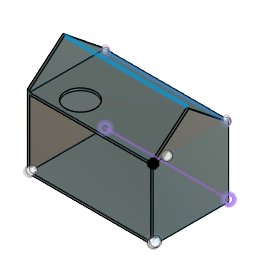
Haus SH (Autodesk Fusion 360 design; units mm, degrees)
part number: 2026-08-06-17-03-33-858
Autodesk Fusion 360 part; units mm, degrees
sketch "Sketch1" plane through (0, 0, 0) normal (0, 0, 1) x (1, 0, 0)
  line L0 (0, 0) -> (275, 0)
  line L1 (275, 0) -> (275, -165)
  line L2 (275, -165) -> (0, -165)
  line L3 (0, -165) -> (0, 0)
  dimension "d1" = 275
  dimension "d2" = 165
  constraint horizontal L0
  constraint vertical L1
  constraint horizontal L2
  constraint vertical L3
  constraint coincident L0.start L3.end
  measures "d1" distance of L0.start L0.end
  measures "d2" distance of L0.start L2.end
extrude "Extrude1" add sketch "Sketch1" along normal blind 5
sketch "Sketch2" plane through (0, 0, 5) normal (0, 0, 1) x (-1, 0, 0)
  line L0 (0, 165) -> (-275, 165)
  line L1 (-275, 165) -> (-275, 0)
  line L2 (-275, 0) -> (0, 0)
  line L3 (0, 0) -> (0, 165)
  line L4 (0, 0) -> (-275, 0)
  line L5 (-275, 0) -> (-275, 5)
  line L6 (-275, 5) -> (0, 5)
  line L7 (0, 5) -> (0, 0)
  line L8 (-275, 0) -> (-270, 0)
  line L9 (-270, 0) -> (-270, 165)
  line L10 (-270, 165) -> (-275, 165)
  line L11 (-275, 165) -> (-275, 0)
  line L12 (-275, 165) -> (0, 165)
  line L13 (0, 165) -> (0, 160)
  line L14 (0, 160) -> (-275, 160)
  line L15 (-275, 160) -> (-275, 165)
  line L16 (0, 0) -> (-5, 0)
  line L17 (-5, 0) -> (-5, 165)
  line L18 (-5, 165) -> (0, 165)
  line L19 (0, 165) -> (0, 0)
  dimension "d5" = 5
  dimension "d6" = 5
  dimension "d7" = 165
  dimension "d8" = 275
  dimension "d9" = 5
  dimension "d10" = 165
  constraint horizontal L4
  constraint vertical L5
  constraint horizontal L6
  constraint vertical L7
  constraint coincident L2.end L3.start
  constraint horizontal L8
  constraint vertical L9
  constraint horizontal L10
  constraint vertical L11
  constraint coincident L1.end L2.start
  constraint horizontal L12
  constraint vertical L13
  constraint horizontal L14
  constraint vertical L15
  constraint coincident L0.end L1.start
  constraint horizontal L16
  constraint vertical L17
  constraint horizontal L18
  constraint vertical L19
  measures "d5" distance of L2.end L6.end
  measures "d6" distance of L1.end L8.end
  measures "d7" distance of L1.end L0.end
  measures "d8" distance of L0.end L0.start
  measures "d9" distance of L0.end L14.end
  measures "d10" distance of L2.end L0.start
sketch "Sketch3" plane through (0, 0, 5) normal (0, 0, 1) x (-1, 0, 0)
extrude "Extrude2" add sketch "Sketch2" along normal blind 150 contours L0 L3 L12 L13 L14 L17 L18 L19 | L3 L6 L14 L17 L19 | L2 L3 L4 L6 L7 L16 L17 L19
sketch "Sketch4" plane through (0, 0, 5) normal (0, 0, 1) x (-1, 0, 0)
  line L0 (-5, 0) -> (-5, 165)
  line L1 (-5, 165) -> (-275, 165)
  line L2 (-275, 165) -> (-275, 0)
  line L3 (-275, 0) -> (-5, 0)
sketch "Sketch5" plane through (0, 0, 5) normal (0, 0, 1) x (-1, 0, 0)
  line L0 (-275, 0) -> (-270, 0)
  line L1 (-270, 0) -> (-270, 165)
  line L2 (-270, 165) -> (-275, 165)
  line L3 (-275, 165) -> (-275, 0)
  line L4 (-5, 0) -> (-5, 165)
  dimension "d13" = 5
  dimension "d14" = 165
  dimension "d15" = 270
  constraint horizontal L0
  constraint vertical L1
  constraint horizontal L2
  constraint vertical L3
  measures "d13" distance of L0.start L0.end
  measures "d14" distance of L0.start L2.end
  measures "d15" distance of L3 L4
extrude "Extrude3" add sketch "Sketch5" along normal blind 150
sketch "Sketch6" plane through (0, 0, 0) normal (0, 1, 0) x (1, 0, 0)
  line L0 (269.7146, -155) -> (269.7146, -150)
  line L1 (4.7146, -150) -> (4.7146, -155)
  line L2 (5, -5) -> (275, -5)
  dimension "d19" = 5
  constraint vertical L0
  constraint vertical L1
  measures "d19" distance of L1.end L1.start
sketch "Sketch7" plane through (0, 0, 5) normal (0, 0, 1) x (-1, 0, 0)
  line L0 (-5.2103, 3.9572, 144.946) -> (-270.2103, 3.9572, 144.946)
  line L1 (-270.2103, 3.9572, 144.946) -> (-270.2103, 3.9573, 149.9988)
  line L2 (-270.2103, 3.9573, 149.9988) -> (-5.2104, 3.9572, 149.946)
  line L3 (-5.2104, 3.9572, 149.946) -> (-5.2103, 3.9572, 144.946)
  line L4 (-275, 165) -> (-275, 160)
  line L5 (-275, 165) -> (-275, 160)
  line L6 (-5, 160) -> (-5, 165)
  line L7 (-5, 0) -> (-275, 0)
  dimension "d21" = 265
  dimension "d22" = 5
  dimension "d25" = 270
  dimension "d26" = 145
  dimension "d27" = 265
  constraint vertical L4
  constraint vertical L5
  constraint vertical L6
  measures "d25" distance of L6.end L4.start
sketch "Sketch8" plane through (0, 0, 0) normal (0, 1, 0) x (1, 0, 0)
  line L0 (5.2103, -149.946) -> (270.2103, -149.946)
  line L1 (5, -5) -> (275, -5)
sketch "Sketch9" plane through (0, 0, 5) normal (0, 0, 1) x (1, 0, 0)
sketch "Sketch10" plane through (275, 0, 0) normal (1, 0, 0) x (0, 1, 0)
  line L0 (-165, 0) -> (0, 0)
  line L1 (0, 0) -> (0, 155)
  line L2 (0, 155) -> (-165, 155)
  line L3 (-165, 155) -> (-165, 0)
  line L4 (-165, 155) -> (0, 155)
  line L5 (0, 155) -> (0, 150)
  line L6 (0, 150) -> (-165, 150)
  line L7 (-165, 150) -> (-165, 155)
  dimension "d29" = 165
  dimension "d30" = 5
  constraint horizontal L4
  constraint vertical L5
  constraint horizontal L6
  constraint vertical L7
  constraint coincident L2.end L3.start
  measures "d29" distance of L2.end L1.end
  measures "d30" distance of L2.end L6.end
extrude "Extrude4" add sketch "Sketch10" against normal blind 275 contours L1 L2 L3 L4 L5 L6 L7
sketch "Sketch11" plane through (0, 0, 0) normal (0, 1, 0) x (1, 0, 0)
sketch "Sketch12" plane through (0, 0, 0) normal (0, 1, 0) x (1, 0, 0)
sketch "Sketch13" plane through (275, 0, 0) normal (1, 0, 0) x (0, 1, 0)
  line L0 (-165, 155) -> (-165, 0)
  line L1 (-165, 0) -> (0, 0)
  line L2 (0, 0) -> (0, 155)
  line L3 (0, 155) -> (-165, 155)
  line L4 (-165, 155) -> (-135, 155) construction
  constraint horizontal L4
  constraint coincident L0.start L3.end
sketch "Sketch14" plane through (275, 0, 0) normal (1, 0, 0) x (0, 1, 0)
  line L0 (-170, 155) -> (-5, 155)
  line L1 (-5, 155) -> (-5, 225)
  line L2 (-5, 225) -> (-170, 225)
  line L3 (-170, 225) -> (-170, 155)
  line L4 (-165, 5) -> (0, 5)
  line L5 (-170, 155) -> (-87.1175, 224.5467)
  line L6 (-170, 155) -> (-61.8046, 155) construction
  line L7 (-87.1175, 224.5467) -> (13.9338, 144.1668)
  line L8 (-87.1175, 224.5467) -> (42.0037, 224.5467) construction
  dimension "d35" = 165
  dimension "d36" = 70
  dimension "d37" = 150
  dimension "d38" = 40
  dimension "d39" = 38.5
  constraint horizontal L0
  constraint vertical L1
  constraint horizontal L2
  constraint vertical L3
  constraint horizontal L6
  constraint horizontal L8
  measures "d35" distance of L0.start L0.end
  measures "d36" distance of L0.start L2.end
  measures "d37" distance of L0 L4
  measures "d38" angle of L5 L6
  measures "d39" angle of L7 L8
extrude "Extrude5" add sketch "Sketch14" against normal blind 5 contours L0 L1 L5 L7
sketch "Sketch15" plane through (0, 0, 155) normal (0, 0, 1) x (-1, 0, 0)
  line L0 (-270, 5) -> (-275, 5)
  line L1 (-275, 5) -> (-275, 0)
  line L2 (-275, 0) -> (0, 0)
  line L3 (0, 0) -> (0, 165)
  line L4 (0, 165) -> (-270, 165)
  line L5 (-270, 165) -> (-270, 5)
sketch "Sketch16" plane through (0, 0, 0) normal (-1, 0, 0) x (0, -1, 0)
  line L0 (0, 155) -> (0, 0)
  line L1 (0, 0) -> (165, 0)
  line L2 (165, 0) -> (165, 155)
  line L3 (165, 155) -> (0, 155)
  line L4 (0, 155) -> (87.0576, 225.2184)
  line L5 (87.0576, 225.2184) -> (165, 159.0254)
  line L6 (165, 159.0254) -> (165, 155)
  constraint coincident L0.start L3.end
  constraint coincident L2.end L3.start
  constraint perpendicular L3 L6
extrude "Extrude6" add sketch "Sketch16" against normal blind 5 contours L3 L4 L5 L6
sketch "Sketch17" plane through (5, 0, 0) normal (1, 0, 0) x (0, 1, 0)
  line L0 (-87.0576, 225.2184) -> (-165, 159.0254)
  line L1 (-165, 159.0254) -> (-165, 155)
  line L2 (-165, 155) -> (0, 155)
  line L3 (0, 155) -> (-87.0576, 225.2184)
sketch "Sketch18" plane through (0, 0, 0) normal (0, 1, 0) x (1, 0, 0)
  line L0 (5, -225.2184, -87.0576) -> (270, -225.2184, -87.0576)
  line L1 (270, -225.2184, -87.0576) -> (270, -220.2184, -87.0576)
  line L2 (270, -220.2184, -87.0576) -> (5, -220.2184, -87.0576)
  line L3 (5, -220.2184, -87.0576) -> (5, -225.2184, -87.0576)
  dimension "d44" = 265
  dimension "d45" = 5
sketch "Sketch19" plane through (275, 0, 0) normal (1, 0, 0) x (0, 1, 0)
  line L0 (-165, 155) -> (-165, 0)
  line L1 (-165, 0) -> (0, 0)
  line L2 (0, 0) -> (0, 155)
  line L3 (0, 155) -> (-5, 155)
  line L4 (-5, 155) -> (-5, 159.2275)
  line L5 (-5, 159.2275) -> (-87.1175, 224.5467)
  line L6 (-87.1175, 224.5467) -> (-170, 155)
  line L7 (-170, 155) -> (-165, 155)
  line L8 (-165, 155) -> (-87, 220)
  line L9 (-87, 220) -> (-46.1419, 187.5)
  line L10 (-46.1419, 187.5) -> (-5, 155)
  constraint coincident L0.start L7.end
  constraint parallel L5 L9
  constraint coincident L3.end L4.start
sketch "Sketch20" plane through (0, 0, 155) normal (0, 0, 1) x (-1, 0, 0)
  circle A0 centre (-75, 123.9573) radius 32.5
  line L0 (-270, 165) -> (-270, 5)
  line L1 (-270.2103, 3.9573) -> (-5.2104, 3.9572)
  dimension "d46" = 65
  dimension "d47" = 195
  dimension "d48" = 120
  measures "d46" diameter of A0
  measures "d47" distance of A0.centre L0
  measures "d48" distance of A0.centre L1
extrude "Extrude7" cut sketch "Sketch20" against normal blind 5
sketch "Sketch21" plane through (275, 0, 0) normal (1, 0, 0) x (0, 1, 0)
sketch "Sketch22" plane through (5, 0, 0) normal (1, 0, 0) x (0, 1, 0)
extrude "Extrude8" cut sketch "Sketch19" against normal blind 150 contours L4 L5 L6 L7 L8 L9 L10
sketch "Sketch23" plane through (0, 0, 0) normal (0, 1, 0) x (1, 0, 0)
equation "d1 = 165 mm + 65 mm + 35 mm + 10 mm"
equation "d2 = 55 mm + 48 mm + 10 mm + 52 mm"
